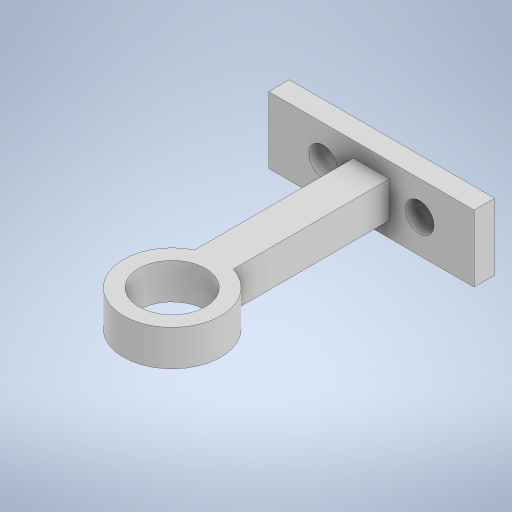
# Autodesk Inventor part: T字形固定件
Saved by Autodesk Inventor 2023 (Build 270158000, 158)
## iProperties
Created: 2024-05-21
Part Number: T字形固定件
Material: 一般
Document SubType Name: Modeling
Designer: anchi_lab
Density: 1 g/cm^3
Appearance: 預設
Author: anchi_lab
Autodesk Inventor part; units mm, degrees
ref_plane "YZ Plane" through (0, 0, 0) normal (1, 0, 0) x (0, 1, 0)
ref_plane "XZ Plane" through (0, 0, 0) normal (0, 1, 0) x (-1, 0, 0)
sketch "草圖1" plane through (0, 0, 0) normal (0, 0, 1) x (1, 0, 0)
  line L0 (-20, 6.5) -> (20, 6.5)
  line L1 (20, 6.5) -> (20, -6.5)
  line L2 (20, -6.5) -> (-20, -6.5)
  line L3 (-20, -6.5) -> (-20, 6.5)
  line L4 (-20, 6.5) -> (20, -6.5) construction
  line L5 (20, 6.5) -> (-20, -6.5) construction
  circle A0 centre (-9.4, 0) radius 2.8
  circle A1 centre (9.4, 0) radius 2.8
  point P0 (0, 0)
  dimension "d0" = 40
  dimension "d1" = 13
  dimension "d2" = 5.6
  dimension "d3" = 5.6
  constraints: 12 end point, 2 centre point, 2 midpoint, 2 parallel, 1 horizontal, 1 perpendicular
  measures "d0" distance of L1.end L2.end
  measures "d1" distance of L0.end L1.end
  measures "d2" diameter of A0
  measures "d3" diameter of A1
extrude "擠出1" add sketch "草圖1" along normal blind 4
sketch "草圖3" plane through (0, 0, 4) normal (0, 0, 1) x (1, 0, 0)
  line L0 (3.5, -3.5) -> (-3.5, -3.5)
  line L1 (-3.5, -3.5) -> (-3.5, 3.5)
  line L2 (-3.5, 3.5) -> (3.5, 3.5)
  line L3 (3.5, 3.5) -> (3.5, -3.5)
  line L4 (3.5, -3.5) -> (-3.5, 3.5) construction
  line L5 (-3.5, -3.5) -> (3.5, 3.5) construction
  point P0 (0, 0)
  dimension "d8" = 7
  dimension "d9" = 7
  constraints: 12 end point, 2 midpoint, 2 parallel, 1 horizontal, 1 perpendicular
  measures "d8" distance of L1.end L2.end
  measures "d9" distance of L0.end L1.end
extrude "擠出2" add sketch "草圖3" along normal blind 33
ref_plane "工作平面2" through (-3.5, 0, 4) normal (0, 1, 0) x (1, 0, 0)
sketch "草圖4" plane through (-3.5, 0, 4) normal (0, 1, 0) x (1, 0, 0)
  circle A0 centre (4.1663, -39.5) radius 9.5
  circle A1 centre (4.1663, -39.5) radius 6.5
  dimension "d14" = 19
  dimension "d15" = 13
  constraints: 2 centre point, 1 coincident
  measures "d14" diameter of A0
  measures "d15" diameter of A1
extrude "擠出3" add sketch "草圖4" along normal mid plane 7
